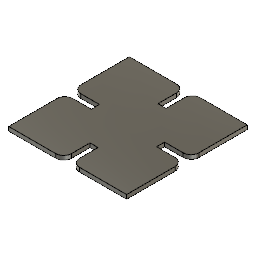
Gara Week 2 assignment v2 (Autodesk Fusion 360 design; units mm, degrees)
Autodesk Fusion 360 part; units mm, degrees
sketch "Sketch1" plane through (0, 0, 0) normal (0, 0, 1) x (1, 0, 0)
  line L0 (0, 46.4728) -> (44.7124, 46.4728)
  line L1 (44.7124, 46.4728) -> (44.7124, 0.7041)
  line L2 (44.7124, 0.7041) -> (0, 0.7041)
  line L3 (0, 0.7041) -> (0, 46.4728)
  line L4 (34.7124, 10.7041) -> (10, 10.7041)
  line L5 (10, 10.7041) -> (10, 36.4728)
  line L6 (10, 36.4728) -> (34.7124, 36.4728)
  line L7 (34.7124, 36.4728) -> (34.7124, 10.7041)
  line L8 (22.3562, 46.4728) -> (22.3562, 0.7041) construction
  line L9 (0, 23.5884) -> (44.7124, 23.5884) construction
  line L10 (0, 22.0884) -> (44.7124, 22.0884)
  line L11 (0, 22.0884) -> (44.7124, 22.0884)
  line L12 (20.8562, 46.4728) -> (20.8562, 0.7041)
  line L13 (0, 25.0884) -> (44.7124, 25.0884)
  line L14 (23.8562, 46.4728) -> (23.8562, 0.7041)
  dimension "d1" = 10
  dimension "d2" = 1.5
  dimension "d3" = 1.5
  constraint horizontal L0
  constraint vertical L1
  constraint horizontal L2
  constraint vertical L3
  constraint midpoint L0 L8.start
  constraint midpoint L2 L8.end
  constraint midpoint L3 L9.start
  constraint midpoint L1 L9.end
  constraint symmetric L11.start L10 L10.start
  constraint symmetric L11.end L10 L10.end
  constraint symmetric L9 L10.start L13.start
  constraint symmetric L9 L10.end L13.end
  constraint symmetric L8 L12.start L14.start
  constraint symmetric L8 L12.end L14.end
extrude "Extrude1" add sketch "Sketch1" along normal blind 1.6 contours L0 L3 L5 L6 L12 L13 | L0 L1 L6 L7 L13 L14 | L5 L6 L12 L13 | L6 L12 L13 L14 | L2 L3 L4 L5 L10 L11 L12 | L5 L10 L11 L12 L13 | L6 L7 L13 L14 | L10 L11 L12 L13 L14 | L4 L5 L10 L11 L12 | L7 L10 L11 L13 L14 | L4 L10 L11 L12 L14 | L1 L2 L4 L7 L10 L11 L14 | L4 L7 L10 L11 L14
fillet "Fillet1" radius 3 5 edges at (0, 22.0884, 0.8) (0, 25.0884, 0.8) (20.8562, 0.7041, 0.8) (23.8562, 0.7041, 0.8) (44.7124, 25.0884, 0.8)
fillet "Fillet2" radius 3 3 edges at (23.8562, 46.4728, 0.8) (20.8562, 46.4728, 0.8) (44.7124, 22.0884, 0.8)
